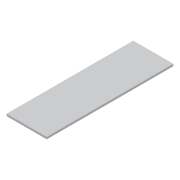
# Autodesk Inventor part: ScaleCompartment_FloorPlate
Saved by Autodesk Inventor 2016 (Build 200138000, 138)
## iProperties
Created: 2014-11-14
Part Number: ScaleCompartment_FloorPlate
Material: Polycarbonat, klar
Document SubType Name: Modeling
Designer: Gero Hofmann
Density: 1.2 g/cm^3
Appearance: Polycarbonat - klar
Author: Gero Hofmann
Autodesk Inventor part; units mm, degrees
ref_plane "YZ Plane" through (0, 0, 0) normal (1, 0, 0) x (0, 1, 0)
ref_plane "XZ Plane" through (0, 0, 0) normal (0, 1, 0) x (-1, 0, 0)
sketch "Skizze1" plane through (0, 0, 0) normal (0, 0, 1) x (1, 0, 0)
  line L0 (95, -300) -> (-95, -300)
  line L1 (-95, -300) -> (-95, 300)
  line L2 (-95, 300) -> (95, 300)
  line L3 (95, 300) -> (95, -300)
  line L4 (95, -300) -> (-95, 300) construction
  line L5 (-95, -300) -> (95, 300) construction
  point P0 (0, 0)
  dimension "d0" = 190
  dimension "d1" = 600
  constraints: 12 end point, 2 midpoint, 2 parallel, 1 horizontal, 1 perpendicular
  measures "d0" distance of L1.end L2.end
  measures "d1" distance of L0.end L1.end
extrude "Extrusion1" add sketch "Skizze1" along normal blind 10
ref_plane "Arbeitsebene1" through (100, -350, 89) normal (0, 0, -1) x (0, 1, 0)
